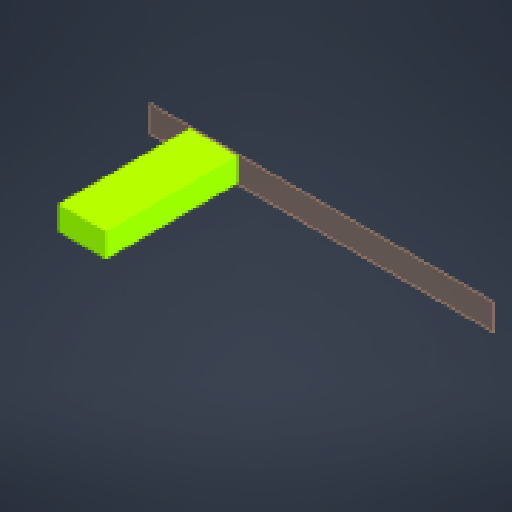
# Autodesk Inventor part: 2x4x(Rename)
Saved by Autodesk Inventor 2027 (Build 310192000, 192)
## iProperties
Created: 2026-08-07
Part Number: 2x4x(Rename)
Material: Generic
Document SubType Name: Modeling
Designer: lucas
Density: 1 g/cm^3
Appearance: Default
Author: lucas
Autodesk Inventor part; units mm, degrees
ref_plane "YZ Plane" through (0, 0, 0) normal (1, 0, 0) x (0, 1, 0)
ref_plane "XZ Plane" through (0, 0, 0) normal (0, 1, 0) x (-1, 0, 0)
ref_plane "XY Plane" through (0, 0, 0) normal (0, 0, 1) x (1, 0, 0)
ref_plane "Work Plane1" through (25.4, -88.9, 0) normal (0, 0, 1) x (1, 0, 0)
sketch "Sketch1" plane through (25.4, -88.9, 0) normal (0, 0, 1) x (1, 0, 0)
  line L0 (-609.6, 50.8) -> (-609.6, 0) projected
  line L1 (-609.6, 0) -> (-508.2062, 0) projected
  line L2 (-609.6, 0) -> (-520.7, 0)
  line L3 (-520.7, 0) -> (-520.7, 38.1)
  line L4 (-520.7, 38.1) -> (-609.6, 38.1)
  line L5 (-609.6, 38.1) -> (-609.6, 0)
  point P0 (-25.4, 88.9)
  point P1 (-609.6, 38.1)
  point P2 (-520.7, 0)
  dimension "d2" = 88.9
  dimension "d3" = 38.1
  constraints: 8 end point, 2 parallel, 1 horizontal, 1 perpendicular
  measures "d2" distance of L3.end L4.end
  measures "d3" distance of L2.end L3.end
extrude "Extrusion1" add sketch "Sketch1" along normal blind 279.4
body "Solid1"
